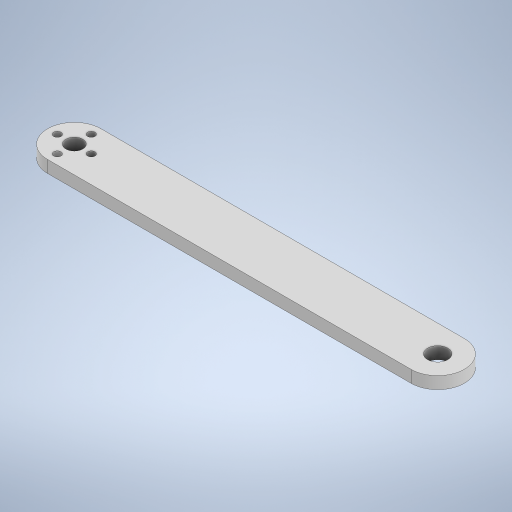
# Autodesk Inventor part: leg1
Saved by Autodesk Inventor 2024 (Build 280153000, 153)
## iProperties
Created: 2023-08-18
Part Number: leg1
Material: 常规
Document SubType Name: Modeling
Designer: wya
Density: 1 g/cm^3
Appearance: 默认
Author: wya
Autodesk Inventor part; units mm, degrees
ref_plane "YZ Plane" through (0, 0, 0) normal (1, 0, 0) x (0, 1, 0)
ref_plane "XZ Plane" through (0, 0, 0) normal (0, 1, 0) x (-1, 0, 0)
ref_plane "XY Plane" through (0, 0, 0) normal (0, 0, 1) x (1, 0, 0)
sketch "草图1" plane through (0, 0, 0) normal (0, 1, 0) x (-1, 0, 0)
  circle A0 centre (0, 0) radius 11
  line L0 (0, 11) -> (-150, 11)
  line L1 (-150, 11) -> (-150, -11)
  line L2 (-150, -11) -> (0, -11)
  line L3 (0, -11) -> (0, 11)
  circle A1 centre (0, 0) radius 3.5
  circle A2 centre (0, 0) radius 7
  circle A3 centre (7, 0) radius 1.525
  circle A4 centre (0, 7) radius 1.525
  circle A5 centre (-7, 0) radius 1.525
  circle A6 centre (0, -7) radius 1.525
  line L4 (7, 0) -> (-7, 0)
  circle A7 centre (-150, 0) radius 11
  circle A8 centre (-150, 0) radius 4.15
  point P0 (0, 0)
  point P1 (0, -11)
  dimension "d1" = 22
  dimension "d0" = 7
  dimension "d2" = 14
  dimension "d3" = 3.05
  dimension "d4" = 3.05
  dimension "d5" = 3.05
  dimension "d6" = 3.05
  dimension "d7" = 150
  dimension "d8" = 8.3
  constraints: 10 end point, 7 centre point, 4 coincident, 4 midpoint, 4 point on circle, 3 horizontal, 2 parallel, 2 point on line, 1 perpendicular, 6 other
  measures "d0" diameter of A1
  measures "d2" diameter of A2
  measures "d3" diameter of A3
  measures "d4" diameter of A4
  measures "d5" diameter of A5
  measures "d6" diameter of A6
  measures "d7" distance between parallel lines of L1 L3
  measures "d8" diameter of A8
extrude "拉伸1" add sketch "草图1" along normal blind 5 contours A0 L3 A6 A2 A3 A4 | L3 A4 A2 A5 A6 A0 | A0 L2 A7 L0 | A7 L1 A8 | L1 A8 A7 | A4 L3 A1 L4 A5 A2 | A2 A5 L4 A1 L3 A6 | A4 A2 A3 L4 A1 L3 | L3 A1 L4 A3 A2 A6
